A1 (Autodesk Fusion 360 design; units mm, degrees)
Autodesk Fusion 360 part; units mm, degrees
sketch "Sketch" plane through (0, 0, 0) normal (0, 0, 1) x (-1, 0, 0)
  line L0 (0, 0) -> (-42, 0)
  line L1 (-42, 66) -> (0, 66)
  line L2 (0, 66) -> (0, 0)
  line L3 (-42, 0) -> (-42, 66)
  line L4 (-12, 54) -> (0, 54)
  line L5 (-12, 66) -> (-12, 54)
  line L6 (0, 54) -> (0, 66)
  line L7 (0, 66) -> (-12, 66)
  line L8 (-30, 66) -> (-30, 54)
  line L9 (-42, 54) -> (-42, 66)
  line L10 (-42, 66) -> (-30, 66)
  line L11 (-30, 54) -> (-42, 54)
  line L12 (-42, 0) -> (-42, 12)
  line L13 (-42, 12) -> (0, 12)
  line L14 (0, 12) -> (0, 0)
  line L15 (0, 0) -> (-42, 0)
  line L16 (0, 54) -> (-12, 66)
  line L17 (-30, 66) -> (-42, 54)
  line L18 (-21, 66) -> (-21, 12)
  line L19 (-21, 12) -> (-27, 12)
  line L20 (-21, 66) -> (-21, 12)
  line L21 (-27, 66) -> (-21, 66)
  line L22 (-27, 12) -> (-27, 66)
  line L23 (-21, 12) -> (-15, 12)
  line L24 (-15, 66) -> (-21, 66)
  line L25 (-15, 12) -> (-15, 66)
  line L26 (-21, 66) -> (-21, 12)
  dimension "d1" = 42
  dimension "d2" = 66
  dimension "d3" = 12
  dimension "d4" = 12
  dimension "d5" = 12
  dimension "d6" = 12
  dimension "d7" = 12
  dimension "d8" = 42
  dimension "d9" = 54
  dimension "d10" = 6
  dimension "d11" = 6
  dimension "d12" = 54
  constraint horizontal L1
  constraint horizontal L0
  constraint vertical L3
  constraint vertical L2
  constraint coincident L0.start L2.end
  constraint horizontal L4
  constraint vertical L6
  constraint horizontal L7
  constraint vertical L5
  constraint horizontal L10
  constraint vertical L8
  constraint horizontal L11
  constraint vertical L9
  constraint vertical L12
  constraint vertical L14
  constraint horizontal L15
  constraint horizontal L13
  constraint midpoint L13 L18.end
  constraint midpoint L1 L18.start
  constraint horizontal L19
  constraint vertical L22
  constraint vertical L20
  constraint horizontal L21
  constraint horizontal L23
  constraint horizontal L24
  constraint vertical L25
  constraint vertical L26
  measures "d1" distance of L0.end L0.start
  measures "d2" distance of L0.start L1.end
  measures "d3" distance of L1.end L4.end
  measures "d4" distance of L1.end L5.start
  measures "d5" distance of L1.start L8.start
  measures "d6" distance of L1.start L9.start
  measures "d7" distance of L0.start L13.end
  measures "d8" distance of L0.start L0.end
  measures "d9" distance of L18.end L18.start
  measures "d10" distance of L18.end L19.end
  measures "d11" distance of L18.end L23.end
  measures "d12" distance of L18.end L18.start
extrude "Extrude1" add sketch "Sketch" along normal blind 12 contours L1 L2 L4 L5 L13 L25 | L1 L3 L8 L11 L13 L22 | L4 L5 L16 | L1 L13 L18 L20 L23 L24 L25 L26 | L8 L11 L17 | L1 L13 L18 L19 L20 L21 L22 L26
extrude "Extrude2" add sketch "Sketch" along normal blind 60 contours L0 L2 L3 L12 L13 L14 L15 L19 L23
fillet "Fillet1" radius 21 2 edges at (42, -6, 60) (0, -6, 60)
extrude "Extrude4" add sketch "Sketch" along normal blind 54 contours L1 L13 L18 L20 L23 L24 L25 L26 | L1 L13 L18 L19 L20 L21 L22 L26
chamfer "Chamfer1" distance 54 distance2 42 1 edges at (21, -66, 54) measured on face at (23, -30, 54)
